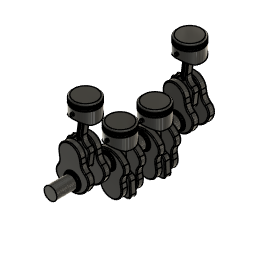
Piston (Autodesk Fusion 360 design; units mm, degrees)
Autodesk Fusion 360 part; units mm, degrees
note: some values were not read from the file. Set by a fixed rule: which face or edge a step refers to.
sketch "Sketch1" plane through (0, 0, 0) normal (0, 1, 0) x (1, 0, 0) in component "piston"
  line L0 (0, 0) -> (40, 0)
  line L1 (40, 0) -> (40, -57)
  line L2 (40, -57) -> (0, -57)
  line L3 (0, -57) -> (0, 0)
  line L4 (40, -50) -> (36, -50)
  line L5 (36, -50) -> (36, -48)
  line L6 (36, -48) -> (40, -48)
  line L7 (40, -48) -> (40, -50)
  line L8 (40, -46) -> (36, -46)
  line L9 (36, -46) -> (36, -44)
  line L10 (36, -44) -> (40, -44)
  line L11 (40, -44) -> (40, -46)
  line L12 (40, -40) -> (36, -40)
  line L13 (36, -40) -> (36, -38)
  line L14 (36, -38) -> (40, -38)
  line L15 (40, -38) -> (40, -40)
  dimension "d3" = 2
  dimension "d4" = 2
  dimension "d5" = 2
  dimension "d6" = 4
  dimension "d7" = 4
  dimension "d8" = 4
  dimension "d9" = 7
  dimension "d10" = 2
  dimension "d11" = 4
  constraint horizontal L0
  constraint vertical L1
  constraint horizontal L2
  constraint vertical L3
  constraint coincident L0.start L3.end
  constraint horizontal L4
  constraint vertical L5
  constraint horizontal L6
  constraint vertical L7
  constraint coincident L1 L4.start
  constraint horizontal L8
  constraint vertical L9
  constraint horizontal L10
  constraint vertical L11
  constraint coincident L1 L8.start
  constraint horizontal L12
  constraint vertical L13
  constraint horizontal L14
  constraint vertical L15
  constraint coincident L1 L12.start
  measures "d3" distance of L4.end L5.end
  measures "d4" distance of L8.end L9.end
  measures "d5" distance of L12.end L13.end
  measures "d6" distance of L4.start L4.end
  measures "d7" distance of L8.start L8.end
  measures "d8" distance of L12.start L12.end
  measures "d9" distance of L2 L4
  measures "d10" distance of L6 L8
  measures "d11" distance of L10 L12
revolve "Revolve1" add sketch "Sketch1" angle 360 about axis through (0, 0, 57) along (0, 0, -1) contours L0 L1 L2 L3 L4 L5 L6 L8 L9 L10 L12 L13 L14 makes body 1 in component "piston"
fillet "Fillet1" radius 5 1 edges at (-37.2931, -14.4646, 57) on bodies 1 in component "piston"
sketch "Sketch2" plane through (0, 0, 0) normal (0, 0, -1) x (1, 0, 0) in component "piston"
  circle A0 centre (0, 0) radius 40
  circle A1 centre (0, 0) radius 35
  dimension "d15" = 70
  constraint coincident A0.centre A1.centre
  measures "d15" diameter of A1
extrude "Extrude1" cut sketch "Sketch2" against normal blind 50 contours A1 bodies 1 in component "piston"
sketch "Sketch3" plane through (0, 0, 0) normal (0, 1, 0) x (1, 0, 0) in component "piston"
  line L0 (-40, 0) -> (40, 0)
  line L1 (-40, -38) -> (40, -38)
  line L2 (0, 0) -> (0, -10)
  arc A0 (-35.5, 0) -> (35.5, 0) centre (0, 52.0459) ccw
  circle A1 centre (0, -24) radius 5
  dimension "d18" = 10
  dimension "d19" = 10
  dimension "d20" = 4.5
  dimension "d21" = 4.5
  dimension "d22" = 24
  constraint coincident L2.start origin
  constraint perpendicular L0 L2
  constraint coincident L0 A0.end
  constraint coincident L0 A0.start
  measures "d18" distance of L2.start L2.end
  measures "d19" diameter of A1
  measures "d20" distance of L0.start A0.start
  measures "d21" distance of L0.end A0.end
  measures "d22" distance of L2.start A1.centre
extrude "Extrude2" cut sketch "Sketch3" along normal mid plane 90 bodies 1 in component "piston"
pattern_linear "00000000-0000-0000-0000-000000000000" [suppressed] in component "pistons"
sketch "Sketch1 (2)" plane through (0, 0, 0) normal (0, 1, 0) x (1, 0, 0) in component "connecting rod"
  circle A0 centre (0, -20) radius 5
  circle A1 centre (0, -20) radius 8.5
  circle A2 centre (0, 105) radius 22.5
  line L0 (-8.5, -20) -> (-8.5, 55)
  line L1 (0, 105) -> (-36, 105)
  line L2 (-36, 105) -> (-36, 80)
  line L3 (-36, 80) -> (-33.5, 80)
  arc A3 (-8.5, 55) -> (-33.5, 80) centre (-33.5, 55) ccw
  line L4 (0, 105) -> (0, 62.6851) construction
  arc A4 (33.5, 80) -> (8.5, 55) centre (33.5, 55) ccw
  line L5 (36, 80) -> (33.5, 80)
  line L6 (36, 105) -> (36, 80)
  line L7 (0, 105) -> (36, 105)
  line L8 (8.5, -20) -> (8.5, 55)
  line L9 (36, 105) -> (-36, 105)
  line L10 (-36, 105) -> (-36, 141)
  line L11 (-36, 141) -> (36, 141)
  line L12 (36, 141) -> (36, 105)
  circle A5 centre (0, -5) radius 4.75
  circle A6 centre (0, 67.5) radius 4.75
  line L13 (4.75, -5) -> (4.75, 67.5)
  line L14 (-4.75, -5) -> (-4.75, 67.5)
  dimension "d29" = 10
  dimension "d30" = 17
  dimension "d31" = 45
  dimension "d32" = 125
  dimension "d33" = 36
  dimension "d34" = 25
  dimension "d35" = 25
  dimension "d36" = 72
  dimension "d37" = 36
  dimension "d38" = 9.5
  dimension "d39" = 9.5
  dimension "d40" = 15
  dimension "d41" = 37.5
  constraint concentric A0 A1
  constraint coincident A1 L0.start
  constraint tangent A1 L0
  constraint vertical L0
  constraint coincident A2.centre L1.start
  constraint horizontal L1
  constraint perpendicular L1 L2
  constraint perpendicular L0 L3
  constraint tangent L3 A3
  constraint tangent L0 A3
  constraint perpendicular L1 L4
  constraint symmetric L0.start L4 L8.start
  constraint symmetric A2.centre L4 L1.start
  constraint symmetric L1.end L4 L6.start
  constraint symmetric L2.end L4 L5.start
  constraint symmetric L3.end L4 A4.start
  constraint symmetric L0.end L4 A4.end
  constraint symmetric A3 L4 A4
  constraint horizontal L9
  constraint vertical L10
  constraint horizontal L11
  constraint vertical L12
  constraint coincident A5 L13.start
  constraint coincident A6 L13.end
  constraint tangent A6 L13
  constraint parallel L8 L13
  constraint coincident A5 L14.start
  constraint coincident A6 L14.end
  constraint tangent A6 L14
  constraint parallel L0 L14
  measures "d29" diameter of A0
  measures "d30" diameter of A1
  measures "d31" diameter of A2
  measures "d32" distance of A0.centre A2.centre
  measures "d33" distance of A2.centre L1.end
  measures "d34" distance of L1.end L2.end
  measures "d35" radius of A3
  measures "d36" distance of L6.start L1.end
  measures "d37" distance of L6.start L11.end
  measures "d38" diameter of A5
  measures "d39" diameter of A6
  measures "d40" distance of A0.centre A5.centre
  measures "d41" distance of A2.centre A6.centre
extrude "Extrude1'" add sketch "Sketch1 (2)" along normal mid plane 20 separate body contours A1 | A1 A2 L0 L1 L2 L3 A3 A4 L5 L6 L7 L8 L9 | A2 L1 L7 L9 L10 L11 L12 makes body 2 in component "connecting rod"
extrude "Extrude2'" add sketch "Sketch1 (2)" along normal mid plane 10 contours A5 | A5 A6 L13 L14 | A6 bodies 2 in component "connecting rod"
fillet "Fillet1'" radius 12.5 4 edges at (-36, 0, -80) (-36, 0, -141) (36, 0, -80) (36, 0, -141) on bodies 2 in component "connecting rod"
fillet "Fillet2" radius 2.5 24 edges at (0, -10, 28.5) (-8.5, -10, -17.5) (-13.6044, -10, -70.1383) (-33.4478, -10, -83.573) (-36, -10, -109.821) (-32.3388, -10, -137.3388) (0, -10, -141) (32.3388, -10, -137.3388) (36, -10, -109.821) (33.4478, -10, -83.573) (13.6044, -10, -70.1383) (8.5, -10, -17.5) (33.4478, 10, -83.573) (36, 10, -109.821) (32.3388, 10, -137.3388) (0, 10, -141) (-32.3388, 10, -137.3388) (-36, 10, -109.821) (-33.4478, 10, -83.573) (-13.6044, 10, -70.1383) (-8.5, 10, -17.5) (0, 10, 28.5) (8.5, 10, -17.5) (13.6044, 10, -70.1383) on bodies 2 in component "connecting rod"
fillet "Fillet3" radius 1.5 16 edges at (0, 5, 9.75) (-4.75, 5, -31.25) (0, 5, -72.25) (4.75, 5, -31.25) (0, 10, 9.75) (-4.75, 10, -31.25) (0, 10, -72.25) (4.75, 10, -31.25) (4.75, -5, -31.25) (0, -5, -72.25) (-4.75, -5, -31.25) (0, -5, 9.75) (4.75, -10, -31.25) (0, -10, -72.25) (-4.75, -10, -31.25) (0, -10, 9.75) on bodies 2 in component "connecting rod"
pattern_linear "00000000-0000-0000-0000-000000000000'" [suppressed] in component "connecting rods"
cylinder "CylinderPrimitive1" add diameter 10 height 90 placed x (1, 0, 0) y (0, 0, -1) z (0, 1, 0) at (135.5905, 0, 45.9526) separate body makes body 3 in component "pin"
fillet "Fillet1''" radius 1.5 2 edges at (130.9289, 0, 44.1445) (130.9289, 90, 47.7606) on bodies 3 in component "pin"
pattern_linear "00000000-0000-0000-0000-000000000000''" [suppressed] in component "pins"
sketch "Sketch1 (3)" plane through (0, 0, 0) normal (0, 1, 0) x (1, 0, 0) in component "crank shaft"
  circle A0 centre (0, 105) radius 22.5
  circle A1 centre (0, 105) radius 35
  circle A2 centre (0, 40.5) radius 20
  circle A3 centre (0, 40.5) radius 25
  arc A4 (-55, 62.5) -> (55, 62.5) centre (0, 62.5) ccw
  line L0 (-35, 105) -> (-35, 62.5)
  line L1 (35, 105) -> (35, 62.5)
  line L2 (-35, 62.5) -> (-55, 62.5)
  line L3 (35, 62.5) -> (55, 62.5)
  dimension "d64" = 70
  dimension "d65" = 110
  dimension "d66" = 40
  dimension "d67" = 50
  dimension "d68" = 42.5
  dimension "d69" = 22
  constraint concentric A0 A1
  constraint concentric A2 A3
  constraint coincident A1 L0.start
  constraint tangent A1 L0
  constraint coincident A1 L1.start
  constraint tangent A1 L1
  measures "d64" diameter of A1
  measures "d65" diameter of A4
  measures "d66" diameter of A2
  measures "d67" diameter of A3
  measures "d68" distance of A0.centre A4.centre
  measures "d69" distance of A4.centre A2.centre
extrude "Extrude1''" add sketch "Sketch1 (3)" along normal blind 20 from surface at 15 separate body contours A0 | A1 | A1 A4 L0 L1 L2 L3 | A2 | A3 makes body 4 in component "crank shaft"
extrude "Extrude2''" add sketch "Sketch1 (3)" along normal blind 20 from surface at 35 contours A2 bodies 4 in component "crank shaft"
extrude "Extrude3" add sketch "Sketch1 (3)" along normal blind 5 from surface at 35 contours A3 bodies 4 in component "crank shaft"
fillet "Fillet1'''" radius 30 2 edges at (-35, 25, -62.5) (35, 25, -62.5) on bodies 4 in component "crank shaft"
fillet "Fillet2'" radius 25 2 edges at (55, 25, -62.5) (-55, 25, -62.5) on bodies 4 in component "crank shaft"
fillet "Fillet3'" radius 2.5 16 edges at (51.987, 35, -55.6375) (37.4915, 35, -78.8142) (35, 35, -97.8921) (0, 35, -140) (-35, 35, -97.8921) (-37.4915, 35, -78.8142) (-51.987, 35, -55.6375) (0, 35, -7.5) (37.4915, 15, -78.8142) (35, 15, -97.8921) (0, 15, -140) (-35, 15, -97.8921) (-37.4915, 15, -78.8142) (-51.987, 15, -55.6375) (0, 15, -7.5) (51.987, 15, -55.6375) on bodies 4 in component "crank shaft"
fillet "Fillet4" radius 1.5 3 edges at (-18.6465, 40, -33.2677) (-23.3082, 40, -31.4596) (-23.3082, 35, -49.5404) on bodies 4 in component "crank shaft"
mirror "Mirror1" about plane through (0, 0, 0) normal (0, 1, 0) of bodies 4 makes body 5 in component "crank shaft"
extrude "Extrude4" add sketch "Sketch1 (3)" along normal mid plane 30 contours A0 bodies 4 5 in component "crank shaft"
pattern_linear "R-Pattern1" count 4 spacing 110 along (0, -1, 0) of bodies 4 makes body 6 at (-26.5501, -95, -58.8431) makes body 7 at (-26.5501, -205, -58.8431) makes body 8 at (-26.5501, -315, -58.8431) in component "crank shaft"
move_body "Move1" bodies 6 7 to x (-1, 0, 0) y (0, 1, 0) z (0, 0, -1) at (0, 0, -81) in component "crank shaft"
combine "Combine1" operation add target body 8 tool bodies 6 7 4 in component "crank shaft"
extrude "Extrude5" add 1 faces at (1.2228, -385, -45.27) along direction (0, -1, 0) blind 50 on bodies 8 bodies 8 in component "crank shaft"
sketch "Sketch1 (4)" plane through (0, -435, 0) normal (0, -1, 0) x (1, 0, 0)
  circle A0 centre (0, -40.5) radius 20
  circle A1 centre (0, -40.5) radius 37.5
  dimension "d97" = 75
  constraint concentric A0 A1
  measures "d97" diameter of A1
extrude "Extrude1'''" add sketch "Sketch1 (4)" against normal blind 25 separate body makes body 9 in component "Component"
sketch "Sketch2 (2)" plane through (0, 0, 148.75) normal (0, 0, 1) x (-1, 0, 0)
  circle A0 centre (0, 335.0024) radius 35
  line L0 (125, 175) -> (-125, 175)
  line L1 (-125, 175) -> (-125, 650)
  line L2 (-125, 650) -> (125, 650)
  line L3 (125, 650) -> (125, 175)
  circle A1 centre (0, 225.0024) radius 40
  circle A2 centre (0, 335.0024) radius 40
  circle A3 centre (0, 445.0024) radius 40
  circle A4 centre (0, 555.0024) radius 40
  constraint horizontal L0
  constraint vertical L1
  constraint horizontal L2
  constraint vertical L3
extrude "Extrude1''''" add sketch "Sketch2 (2)" along normal blind 25 separate body contours L0 L1 L2 L3 makes body 10 in component "Component'"
component "pistons" placed x (1, 0, 0) y (0, 1, 0) z (0, 0, 1) at (0, 0, 0)
component "connecting rods" placed x (1, 0, 0) y (0, 1, 0) z (0, 0, 1) at (0, 0, 0)
component "pins" placed x (1, 0, 0) y (0, 1, 0) z (0, 0, 1) at (0, 0, 0)
component "crank shaft" placed x (1, 0, 0) y (0, 1, 0) z (0, 0, 1) at (0, -225, -33.25)
component "Component" placed x (1, 0, 0) y (0, 1, 0) z (0, 0, 1) at (0, 0, 0)
component "Component'" placed x (1, 0, 0) y (0, 1, 0) z (0, 0, 1) at (0, 0, 0)
component "piston" placed x (1, 0, 0) y (0, 1, 0) z (0, 0, 1) at (0, -335.0024, 91.75) in component "pistons"
component "piston" placed x (1, 0, 0) y (0, 1, 0) z (0, 0, 1) at (0, -445.0024, 91.75) in component "pistons"
component "piston" placed x (1, 0, 0) y (0, 1, 0) z (0, 0, 1) at (0, -225.0024, -37.25) in component "pistons"
component "piston" placed x (1, 0, 0) y (0, 1, 0) z (0, 0, 1) at (0, -555.0024, -37.25) in component "pistons"
component "connecting rod" placed x (1, 0, 0) y (0, 1, 0) z (0, 0, 1) at (0, -225, -33.25) in component "connecting rods"
component "connecting rod" placed x (1, 0, 0) y (0, 1, 0) z (0, 0, 1) at (0, -335, 95.75) in component "connecting rods"
component "connecting rod" placed x (1, 0, 0) y (0, 1, 0) z (0, 0, 1) at (0, -445, 95.75) in component "connecting rods"
component "connecting rod" placed x (1, 0, 0) y (0, 1, 0) z (0, 0, 1) at (0, -555, -33.25) in component "connecting rods"
component "pin" placed x (1, 0, 0) y (0, 1, 0) z (0, 0, 1) at (-135.5905, -380, 69.7974) in component "pins"
component "pin" placed x (1, 0, 0) y (0, 1, 0) z (0, 0, 1) at (-135.5905, -270, -59.2026) in component "pins"
component "pin" placed x (1, 0, 0) y (0, 1, 0) z (0, 0, 1) at (-135.5905, -490, 69.7974) in component "pins"
component "pin" placed x (1, 0, 0) y (0, 1, 0) z (0, 0, 1) at (-135.5905, -600, -59.2026) in component "pins"
